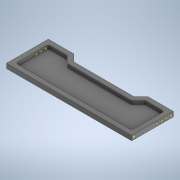
# Autodesk Inventor part: Cockpit_battery_back_door
Saved by Autodesk Inventor 2022.3 (Build 263350000, 350)
## iProperties
Part Number: Cockpit_battery_back_door
Material: アセタール樹脂、黒
Document SubType Name: Modeling
Designer: Masato Kubotera
Density: 1.425 g/cm^3
Appearance: 滑らか - 黒
Description: POM T5
Mass: 40.5621 g
Surface Area: 135.491 cm^2
Volume: 28.4646 cm^3
Author: Masato Kubotera
Autodesk Inventor part; units mm, degrees
ref_plane "XZ Plane" through (0, 0, 0) normal (0, 1, 0) x (-1, 0, 0)
ref_plane "XY Plane" through (0, 0, 0) normal (0, 0, 1) x (1, 0, 0)
derived "Cockpit_side_frame.ipt"
sketch "スケッチ2" plane through (0, 0, 0) normal (0, 1, 0) x (-1, 0, 0)
  line L0 (-23.5, -22.5) -> (-28.5, -27.5)
  line L1 (-28.5, -27.5) -> (-28.5, -91)
  line L2 (-28.5, -91) -> (-23.5, -96)
  line L3 (-23.5, -96) -> (34.25, -96)
  line L4 (36.25, -98) -> (36.25, -128.5)
  line L5 (36.25, -128.5) -> (46.25, -138.5)
  line L6 (46.25, -138.5) -> (86.5, -138.5)
  line L7 (91.5, -133.5) -> (91.5, -20)
  line L8 (91.5, -20) -> (89, -17.5)
  line L9 (89, -17.5) -> (83.25, -17.5)
  line L10 (83.25, -17.5) -> (83.25, -21.0151)
  line L11 (81.7651, -22.5) -> (76.8599, -22.5)
  line L12 (75.375, -21.0151) -> (75.375, -17.5)
  line L13 (75.375, -17.5) -> (60.375, -17.5)
  line L14 (60.375, -17.5) -> (60.375, -21.0151)
  line L15 (58.8901, -22.5) -> (-23.5, -22.5)
  line L16 (-25.25, -25) -> (-20.25, -25) construction
  line L17 (-20.25, -25) -> (-20.25, -93.5) construction
  line L18 (-20.25, -93.5) -> (-25.25, -93.5) construction
  line L19 (-25.25, -93.5) -> (-25.25, -25) construction
  line L20 (-26, -25) -> (-25.25, -25) construction
  line L21 (-25.25, -93.5) -> (-26, -93.5) construction
  line L22 (-26, -93.5) -> (-26, -25) construction
  line L23 (-20.25, -93.5) -> (83.25, -93.5) construction
  line L24 (-20.25, -88.5) -> (83.25, -88.5) construction
  line L25 (83.25, -22.5) -> (83.25, -90) construction
  line L26 (83.25, -90) -> (88.25, -90) construction
  line L27 (88.25, -90) -> (88.25, -22.5) construction
  line L28 (83.25, -88.5) -> (83.25, -93.5) construction
  line L29 (83.25, -91) -> (88.25, -91) construction
  line L30 (88.25, -91) -> (88.25, -136) construction
  line L31 (83.25, -91) -> (83.25, -136) construction
  line L32 (83.25, -136) -> (88.25, -136) construction
  line L33 (38.75, -131) -> (38.75, -93.5) construction
  line L34 (43.75, -93.5) -> (43.75, -131) construction
  line L35 (38.75, -131) -> (43.75, -131) construction
  line L36 (41.25, -131) -> (41.25, -93.5) construction
  line L37 (43.75, -131) -> (81.25, -131) construction
  line L38 (81.25, -131) -> (81.25, -136) construction
  line L39 (81.25, -136) -> (43.75, -136) construction
  line L40 (43.75, -133.5) -> (81.25, -133.5) construction
  line L41 (85.75, -91) -> (85.75, -136) construction
  circle A0 centre (85.75, -133.5) radius 2.975
  arc A1 (83.25, -131) -> (88.25, -131) centre (85.75, -133.5) ccw construction
  line L42 (83.25, -91) -> (-20.25, -91) construction
  line L43 (41.25, -112.25) -> (43.75, -112.25) construction
  line L44 (62.5, -131) -> (62.5, -133.5) construction
  line L45 (41.2, -116.8151) -> (41.2, -107.6849)
  line L46 (43.8, -108.3) -> (43.8, -116.2)
  line L47 (43.8, -118.3) -> (41.2, -106.2) construction
  line L48 (41.2, -118.3) -> (43.8, -106.2) construction
  line L49 (58.55, -130.95) -> (66.45, -130.95)
  line L50 (67.0651, -133.55) -> (57.9349, -133.55)
  line L51 (56.45, -130.95) -> (68.55, -133.55) construction
  line L52 (68.55, -130.95) -> (56.45, -133.55) construction
  line L53 (41.25, -106.25) -> (43.75, -106.25) construction
  line L54 (41.25, -118.25) -> (43.75, -118.25) construction
  arc A2 (42.6849, -106.2) -> (41.2, -107.6849) centre (41.9425, -106.9425) ccw
  arc A3 (43.8, -108.3) -> (43.8, -106.2) centre (43.8, -107.25) ccw
  arc A4 (41.2, -116.8151) -> (42.6849, -118.3) centre (41.9425, -117.5575) ccw
  arc A5 (43.8, -118.3) -> (43.8, -116.2) centre (43.8, -117.25) ccw
  line L55 (56.5, -133.5) -> (56.5, -131) construction
  line L56 (68.5, -131) -> (68.5, -133.5) construction
  arc A6 (56.45, -132.0651) -> (57.9349, -133.55) centre (57.1925, -132.8075) ccw
  arc A7 (58.55, -130.95) -> (56.45, -130.95) centre (57.5, -130.95) ccw
  arc A8 (67.0651, -133.55) -> (68.55, -132.0651) centre (67.8075, -132.8075) ccw
  arc A9 (68.55, -130.95) -> (66.45, -130.95) centre (67.5, -130.95) ccw
  line L57 (56.45, -132.0651) -> (56.45, -130.95)
  line L58 (68.55, -130.95) -> (68.55, -132.0651)
  line L59 (42.6849, -106.2) -> (43.8, -106.2)
  line L60 (43.8, -118.3) -> (42.6849, -118.3)
  circle A10 centre (48.75, -133.5) radius 1.6
  line L61 (88.25, -22.5) -> (88.25, -17.5) construction
  line L62 (89, -17.5) -> (89, -90) construction
  line L63 (89, -90) -> (88.25, -90) construction
  line L64 (-13.5, -82.5) -> (-13.5, -61)
  arc A11 (-13.5, -82.5) -> (-11.5, -84.5) centre (-11.5, -82.5) ccw
  line L65 (45.5, -84.5) -> (-11.5, -84.5)
  arc A12 (45.5, -84.5) -> (47.5, -82.5) centre (45.5, -82.5) ccw
  line L66 (47.5, -61) -> (47.5, -82.5)
  arc A13 (47.5, -61) -> (45.5, -59) centre (45.5, -61) ccw
  line L67 (-11.5, -59) -> (45.5, -59)
  arc A14 (-11.5, -59) -> (-13.5, -61) centre (-11.5, -61) ccw
  line L68 (31.5, -88.5) -> (31.5, -91) construction
  line L69 (85.75, -22.5) -> (85.75, -90) construction
  circle A15 centre (85.75, -31.25) radius 1.6
  circle A16 centre (85.75, -31.25) radius 3
  circle A17 centre (85.75, -81.25) radius 3
  circle A18 centre (85.75, -81.25) radius 1.6
  line L70 (88.25, -22.5) -> (83.25, -22.5) construction
  arc A19 (88.25, -91) -> (83.25, -91) centre (85.75, -133.5) ccw construction
  circle A20 centre (48.75, -133.5) radius 3
  circle A21 centre (41.25, -98.5) radius 1.6
  circle A22 centre (41.25, -98.5) radius 3
  line L71 (10.55, -88.5) -> (10.55, -91) construction
  line L72 (52.45, -88.5) -> (52.45, -91) construction
  line L73 (51.0151, -91.05) -> (11.9849, -91.05)
  line L74 (10.5, -89.5651) -> (10.5, -88.45)
  line L75 (12.6, -88.45) -> (50.4, -88.45)
  line L76 (52.5, -88.45) -> (52.5, -89.5651)
  line L77 (52.5, -91.05) -> (10.5, -88.45) construction
  line L78 (10.5, -91.05) -> (52.5, -88.45) construction
  arc A23 (12.6, -88.45) -> (10.5, -88.45) centre (11.55, -88.45) ccw
  arc A24 (10.5, -89.5651) -> (11.9849, -91.05) centre (11.2425, -90.3075) ccw
  arc A25 (51.0151, -91.05) -> (52.5, -89.5651) centre (51.7575, -90.3075) ccw
  arc A26 (52.5, -88.45) -> (50.4, -88.45) centre (51.45, -88.45) ccw
  line L79 (-20.25, -31) -> (83.25, -31) construction
  line L80 (83.25, -26) -> (-20.25, -26) construction
  line L81 (-20.25, -26) -> (-20.25, -31) construction
  line L82 (-20.25, -28.5) -> (83.25, -28.5) construction
  line L83 (31.5, -31) -> (31.5, -26) construction
  line L84 (11.9849, -31.05) -> (51.0151, -31.05)
  arc A27 (10.5, -29.5651) -> (11.9849, -31.05) centre (11.2425, -30.3075) ccw
  arc A28 (51.0151, -31.05) -> (52.5, -29.5651) centre (51.7575, -30.3075) ccw
  line L85 (10.55, -31) -> (10.55, -26) construction
  line L86 (52.45, -26) -> (52.45, -31) construction
  circle A29 centre (6.5, -28.5) radius 1.6
  circle A30 centre (6.5, -28.5) radius 3
  line L87 (-26, -59.25) -> (-25.25, -59.25) construction
  line L88 (-22.75, -25) -> (-22.75, -93.5) construction
  arc A31 (58.8901, -22.5) -> (60.375, -21.0151) centre (59.6325, -21.7575) ccw
  arc A32 (75.375, -21.0151) -> (76.8599, -22.5) centre (76.1175, -21.7575) ccw
  line L89 (56.4375, -22.5) -> (56.4375, -17.5) construction
  line L90 (79.3125, -22.5) -> (79.3125, -17.5) construction
  circle A33 centre (-22.75, -31.75) radius 1.6
  circle A34 centre (-22.75, -31.75) radius 3
  circle A35 centre (-22.75, -86.75) radius 1.6
  circle A36 centre (-22.75, -86.75) radius 3
  line L91 (60.375, -22.5) -> (75.375, -22.5)
  line L92 (52.5, -17.5) -> (52.5, -22.5) construction
  circle A37 centre (85.75, -98.5) radius 1.475
  circle A38 centre (85.75, -103.5) radius 1.475
  circle A39 centre (85.75, -108.5) radius 1.475
  line L93 (59.5, -88.5) -> (78.75, -88.5)
  line L94 (80.75, -90.5) -> (80.75, -126.5)
  line L95 (78.75, -128.5) -> (48.25, -128.5)
  line L96 (46.25, -126.5) -> (46.25, -110)
  arc A40 (46.25, -126.5) -> (48.25, -128.5) centre (48.25, -126.5) ccw
  arc A41 (78.75, -128.5) -> (80.75, -126.5) centre (78.75, -126.5) ccw
  arc A42 (80.75, -90.5) -> (78.75, -88.5) centre (78.75, -90.5) ccw
  arc A43 (36.25, -98) -> (34.25, -96) centre (34.25, -98) ccw
  circle A44 centre (-13.5, -55) radius 1.75
  circle A45 centre (-13.5, -55) radius 2
  line L97 (23.9, -49.9425) -> (10.1, -49.9425) construction
  line L98 (10.1, -49.9425) -> (10.1, -40.7425) construction
  line L99 (10.1, -40.7425) -> (23.9, -40.7425) construction
  line L100 (23.9, -40.7425) -> (23.9, -49.9425) construction
  line L101 (23.9, -49.9425) -> (10.1, -40.7425) construction
  line L102 (10.1, -49.9425) -> (23.9, -40.7425) construction
  line L103 (9.45, -40.0425) -> (24.55, -40.0425) construction
  line L104 (24.55, -40.0425) -> (24.55, -50.6425) construction
  line L105 (24.55, -50.6425) -> (9.45, -50.6425) construction
  line L106 (9.45, -50.6425) -> (9.45, -40.0425) construction
  line L107 (9.45, -40.0425) -> (24.55, -50.6425) construction
  line L108 (24.55, -40.0425) -> (9.45, -50.6425) construction
  line L109 (10.8849, -39.9925) -> (23.1151, -39.9925)
  line L110 (24.6, -41.4774) -> (24.6, -49.2075)
  line L111 (24.6, -50.6925) -> (9.4, -39.9925) construction
  line L112 (9.4, -50.6925) -> (24.6, -39.9925) construction
  line L113 (23.95, -49.9925) -> (10.05, -40.6925) construction
  line L114 (10.05, -49.9925) -> (23.95, -40.6925) construction
  arc A46 (10.8849, -39.9925) -> (9.4, -41.4774) centre (10.1425, -40.7349) ccw
  arc A47 (11.5349, -40.6925) -> (10.05, -42.1774) centre (10.7925, -41.4349) ccw
  line L115 (9.4, -45.3425) -> (24.6, -45.3425) construction
  line L116 (17, -39.9925) -> (17, -50.6925) construction
  arc A48 (24.6, -41.4774) -> (23.1151, -39.9925) centre (23.8575, -40.7349) ccw
  arc A49 (23.95, -42.1774) -> (22.4651, -40.6925) centre (23.2075, -41.4349) ccw
  arc A50 (10.05, -48.5075) -> (11.5349, -49.9925) centre (10.7925, -49.25) ccw
  arc A51 (9.4, -49.2075) -> (10.8849, -50.6925) centre (10.1425, -49.95) ccw
  arc A52 (22.4651, -49.9925) -> (23.95, -48.5075) centre (23.2075, -49.25) ccw
  arc A53 (23.1151, -50.6925) -> (24.6, -49.2075) centre (23.8575, -49.95) ccw
  line L117 (11.5349, -40.6925) -> (22.4651, -40.6925)
  line L118 (23.95, -42.1774) -> (23.95, -48.5075)
  line L119 (9.4, -49.2075) -> (9.4, -41.4774)
  line L120 (10.05, -48.5075) -> (10.05, -42.1774)
  line L121 (22.4651, -49.9925) -> (11.5349, -49.9925)
  line L122 (23.1151, -50.6925) -> (10.8849, -50.6925)
  line L123 (-13.5, -71.75) -> (47.5, -71.75) construction
  line L124 (85.75, -56.25) -> (88.25, -56.25) construction
  line L125 (85.7, -69.2) -> (85.7, -43.3)
  line L126 (88.3049, -71.3569) -> (85.7, -41.2) construction
  line L127 (85.7, -71.3) -> (88.3, -41.2) construction
  arc A54 (85.7, -41.2) -> (85.7, -43.3) centre (85.7, -42.25) ccw
  arc A55 (88.3, -42.6849) -> (86.8151, -41.2) centre (87.5575, -41.9425) ccw
  arc A56 (85.7, -69.2) -> (85.7, -71.3) centre (85.7, -70.25) ccw
  arc A57 (86.8151, -71.3) -> (88.3, -69.8151) centre (87.5575, -70.5575) ccw
  line L128 (85.75, -41.25) -> (88.25, -41.25) construction
  line L129 (85.75, -71.25) -> (88.25, -71.25) construction
  line L130 (88.3, -42.6849) -> (88.3, -69.8151)
  line L131 (88.3, -66.8652) -> (88.3, -69.8151)
  line L132 (86.8151, -71.3) -> (85.7, -71.3)
  line L133 (85.7, -41.2) -> (86.8151, -41.2)
  line L134 (86.5, -138.5) -> (91.5, -133.5)
  arc A58 (81.7651, -22.5) -> (83.25, -21.0151) centre (82.5075, -21.7575) ccw
  circle A59 centre (85.75, -93.5) radius 2
  circle A60 centre (85.75, -93.5) radius 4 construction
  arc A61 (-13.5, -49) -> (-11.5, -51) centre (-11.5, -49) ccw construction
  line L135 (45.5, -51) -> (-11.5, -51) construction
  arc A62 (45.5, -51) -> (47.5, -49) centre (45.5, -49) ccw construction
  line L136 (10.5, -29.5651) -> (10.5, -22.5)
  line L137 (52.5, -29.5651) -> (52.5, -22.5)
  line L138 (67.875, -17.5) -> (67.875, -22.5) construction
  line L139 (52.5, -17.5) -> (83.25, -17.5) construction
  line L140 (43.75, -131) -> (43.75, -136) construction
  line L141 (57.5, -22.5) -> (57.5, -103) construction
  line L142 (57.5, -103) -> (52.5, -108) construction
  line L143 (-23.5, -108) -> (52.5, -108) construction
  line L144 (57.5, -90.5) -> (57.5, -102.1716)
  line L145 (56.9142, -103.5858) -> (53.0858, -107.4142)
  line L146 (51.6716, -108) -> (48.25, -108)
  arc A63 (59.5, -88.5) -> (57.5, -90.5) centre (59.5, -90.5) ccw
  arc A64 (56.9142, -103.5858) -> (57.5, -102.1716) centre (55.5, -102.1716) ccw
  arc A65 (51.6716, -108) -> (53.0858, -107.4142) centre (51.6716, -106) ccw
  arc A66 (48.25, -108) -> (46.25, -110) centre (48.25, -110) ccw
  point P0 (0, 0)
  point P1 (-25.7227, -96)
  point P2 (-23.5, -22.5)
  point P3 (42.5, -112.25)
  point P4 (62.5, -132.25)
  point P5 (31.5, -89.75)
  point P6 (31.5, -28.5)
  point P7 (52.5, -22)
  point P8 (46.25, -108)
  point P9 (57.5, -88.5)
  point P10 (17, -45.3425)
  point P11 (17, -45.3425)
  point P12 (87, -56.25)
  point P13 (17, -51)
  point P14 (10.5, -31.05)
  dimension "d1" = 88.25
  dimension "d2" = 5
  measures "d1" distance from line of L30 point (0, 0)
  measures "d2" distance of L31.end L30.end
ref_plane "作業平面1" through (-88.25, 0, 0) normal (1, 0, 0) x (0, 1, 0)
sketch "スケッチ3" plane through (-88.25, 0, 0) normal (1, 0, 0) x (0, 1, 0)
  line L0 (0, -91) -> (0, -136)
  line L1 (0, -136) -> (-135, -136)
  line L2 (-135, -136) -> (-135, -91)
  line L3 (-67.5, -98.5) -> (-67.5, -136) construction
  line L4 (0, -113.5) -> (-135, -113.5) construction
  line L5 (-130, -98) -> (-130, -129)
  line L6 (-128, -131) -> (-7, -131)
  line L7 (-5, -129) -> (-5, -98)
  line L8 (-7, -96) -> (-24.6005, -96)
  line L9 (-26.0147, -96.5858) -> (-32.3431, -102.9142)
  line L10 (-33.7574, -103.5) -> (-101.2426, -103.5)
  line L11 (-102.6569, -102.9142) -> (-108.9853, -96.5858)
  line L12 (-110.3995, -96) -> (-128, -96)
  line L13 (-106.9142, -91.5858) -> (-100.5858, -97.9142)
  line L14 (-34.4142, -97.9142) -> (-28.0858, -91.5858)
  line L15 (-135, -91) -> (-108.3284, -91)
  line L16 (-26.6716, -91) -> (0, -91)
  line L17 (-99.1716, -98.5) -> (-35.8284, -98.5)
  arc A0 (-128, -96) -> (-130, -98) centre (-128, -98) ccw
  arc A1 (-130, -129) -> (-128, -131) centre (-128, -129) ccw
  arc A2 (-7, -131) -> (-5, -129) centre (-7, -129) ccw
  arc A3 (-5, -98) -> (-7, -96) centre (-7, -98) ccw
  arc A4 (-24.6005, -96) -> (-26.0147, -96.5858) centre (-24.6005, -98) ccw
  arc A5 (-33.7574, -103.5) -> (-32.3431, -102.9142) centre (-33.7574, -101.5) ccw
  arc A6 (-102.6569, -102.9142) -> (-101.2426, -103.5) centre (-101.2426, -101.5) ccw
  arc A7 (-108.9853, -96.5858) -> (-110.3995, -96) centre (-110.3995, -98) ccw
  arc A8 (-106.9142, -91.5858) -> (-108.3284, -91) centre (-108.3284, -93) ccw
  arc A9 (-100.5858, -97.9142) -> (-99.1716, -98.5) centre (-99.1716, -96.5) ccw
  arc A10 (-35.8284, -98.5) -> (-34.4142, -97.9142) centre (-35.8284, -96.5) ccw
  arc A11 (-26.6716, -91) -> (-28.0858, -91.5858) centre (-26.6716, -93) ccw
  point P0 (0, 0)
  point P1 (-27.5, -91)
  point P2 (-107.5, -91)
  dimension "d4" = 135
  dimension "d22" = 5
  dimension "d25" = 5
  dimension "d26" = 80
  dimension "d28" = 5
  dimension "d31" = 5
  dimension "d32" = 2
  dimension "d33" = 5
  dimension "d34" = 7.5
  dimension "d35" = 45
  constraints: 36 end point, 24 point on circle, 24 tangent, 12 centre point, 11 equal radius, 7 parallel, 6 perpendicular, 4 point on line, 3 horizontal, 3 midpoint, 2 coincident, 1 collinear, 4 other
  measures "d4" distance of L2.end L0.start
  measures "d22" distance between parallel lines of L14 L9
  measures "d25" distance between parallel lines of L0 L7
  measures "d26" distance of point (-107.5, -91) point (-27.5, -91)
  measures "d28" distance between parallel lines of L1 L6
  measures "d31" distance between parallel lines of L8 L16
  measures "d32" radius of A0
  measures "d33" distance between parallel lines of L10 L17
  measures "d34" distance between parallel lines of L15 L17
  measures "d35" angle of L14 L16
extrude "押し出し1" add sketch "スケッチ3" along normal blind 5
hole "穴1" at (28.5, 0, -27.5) at (25.7227, 0, -96) at (23.5, 0, -22.5) at (-52.5, 0, -22) at (13.5, 0, -55) at (-85.75, 0, -98.5) at (-85.75, 0, -103.5) at (-85.75, 0, -108.5) direction (0, -1, 0) diameter 2.9 depth 5 tip angle 118
hole "穴2" at (-85.75, 0, -133.5) at (-85.75, 0, -93.5) direction (0, -1, 0) diameter 3.2 depth 8
ref_plane "作業平面2" through (-88.25, -121.6642, -91) normal (0, 1, 0) x (1, 0, 0)
ref_plane "作業平面3" through (-88.25, -67.5, -136) normal (0, 1, 0) x (1, 0, 0)
mirror "ミラー1" about plane through (-88.25, -67.5, -136) normal (0, 1, 0) of "穴2", "穴1"
extrude "押し出し2" add sketch "スケッチ3" along normal blind 1 contours A0 L12 A7 L11 A6 L10 A5 L9 A4 L8 A3 L7 A2 L6 A1 L5
equation "\"d22\" = d31"
equation "\"d25\" = d31"
equation "\"d28\" = d31"
equation "\"d33\" = d31"
equation "\"d5\" = d2"
equation "\"d3\" = -d1"
